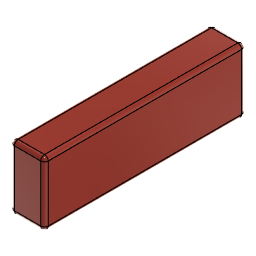
kypom 2cell 2200nAh (Autodesk Fusion 360 design; units mm, degrees)
Autodesk Fusion 360 part; units mm, degrees
sketch "スケッチ1" plane through (0, 0, 0) normal (0, 0, 1) x (1, 0, 0)
  line L0 (0, 0) -> (18, 0)
  line L1 (18, 0) -> (18, 107)
  line L2 (18, 107) -> (0, 107)
  line L3 (0, 107) -> (0, 0)
  dimension "d1" = 18
  dimension "d2" = 107
  constraint horizontal L0
  constraint vertical L1
  constraint horizontal L2
  constraint vertical L3
  constraint coincident L0.start L3.end
  measures "d1" distance of L0.start L0.end
  measures "d2" distance of L0.start L2.end
extrude "押し出し1" add sketch "スケッチ1" along normal blind 34
fillet "フィレット1" radius 2 12 edges at (0, 53.5, 34) (18, 53.5, 34) (9, 107, 34) (9, 0, 34) (18, 0, 17) (18, 107, 17) (18, 53.5, 0) (0, 107, 17) (9, 107, 0) (0, 53.5, 0) (9, 0, 0) (0, 0, 17)
